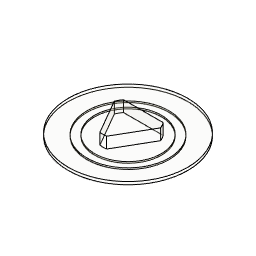
亚克力2 v18 v1 (Autodesk Fusion 360 design; units mm, degrees)
Autodesk Fusion 360 part; units mm, degrees
sketch "草图1" plane through (0, 0, 0) normal (0, 0, 1) x (1, 0, 0)
  arc A0 (-2.4024, -17.839) -> (2.4024, -17.839) centre (0, 0) ccw
  line L0 (0, 0) -> (0, -48) construction
  line L1 (14.2478, 11) -> (-14.2478, 11)
  line L2 (2.4024, -17.839) -> (16.6502, 6.839)
  arc A1 (-14.2478, 11) -> (-16.6502, 6.839) centre (0, 0) ccw
  line L3 (-16.6502, 6.839) -> (-2.4024, -17.839)
  arc A2 (16.6502, 6.839) -> (14.2478, 11) centre (0, 0) ccw
  circle A3 centre (0, 0) radius 43
  constraint coincident A0.centre L0.start
  constraint vertical L0
extrude "拉伸1" add sketch "草图1" against normal blind 2 contours A0 L1 L2 A1 L3 A2 | A3 makes body 1
extrude "拉伸2" add sketch "草图1" along normal blind 8 contours A0 L1 L2 A1 L3 A2 bodies 1
copy_body "实体->零部件1" bodies 1 removing the originals makes body 2 in component "亚克力2"
sketch "草图2" plane through (0, 0, -2) normal (0, 0, -1) x (1, 0, 0)
  circle A0 centre (0, 0) radius 43
  circle A1 centre (0, 0) radius 29.5
  circle A2 centre (0, 0) radius 24
  dimension "d11" = 59
  dimension "d12" = 48
  constraint coincident A0.centre A1.centre
  measures "d11" diameter of A1
  measures "d12" diameter of A2
extrude "拉伸1'" cut sketch "草图2" against normal blind 1 contours A1 bodies 2 in component "亚克力2"
component "亚克力2" placed x (1, 0, 0) y (0, 1, 0) z (0, 0, 1) at (0, 0, 0)
